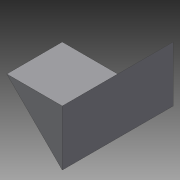
# Autodesk Inventor part: test_part_2
Saved by Autodesk Inventor 2015 (Build 190159000, 159)
## iProperties
Created: 2015-04-25
Part Number: test_part_2
Material: Generic
Document SubType Name: Modeling
Designer: Drew
Density: 1 g/cm^3
Appearance: Default
Author: Drew
Autodesk Inventor part; units mm, degrees
ref_plane "YZ Plane" through (0, 0, 0) normal (1, 0, 0) x (0, 1, 0)
ref_plane "XZ Plane" through (0, 0, 0) normal (0, 1, 0) x (-1, 0, 0)
ref_plane "XY Plane" through (0, 0, 0) normal (0, 0, 1) x (1, 0, 0)
sketch "Sketch1" plane through (0, 0, 0) normal (0, 0, 1) x (1, 0, 0)
  line L0 (0, 0) -> (0, 25.4)
  line L1 (0, 25.4) -> (-25.4, 0)
  line L2 (-25.4, 0) -> (0, 0)
  dimension "d0" = 45
  dimension "d1" = 45
  dimension "d2" = 25.4
  constraints: 6 end point, 1 perpendicular, 1 vertical
  measures "d0" angle of L0 L1
  measures "d1" angle of L2 L1
  measures "d2" distance of L1.end L0.start
extrude "Extrusion1" add sketch "Sketch1" along normal blind 25.4
sketch "Sketch2" plane through (0, 0, 25.4) normal (0, 0, 1) x (1, 0, 0)
  line L0 (0, 0) -> (-25.4, 25.4)
  line L1 (-25.4, 25.4) -> (0, 25.4)
  line L2 (0, 0) -> (0, 25.4) projected
  line L3 (-25.4, 0) -> (-25.4, 25.4)
  dimension "d5" = 25.4
  constraints: 6 end point, 1 perpendicular, 1 vertical
  measures "d5" distance of L0.end L1.end
extrude "Extrusion2" add sketch "Sketch2" along normal blind 25.4
body "Solid1"
